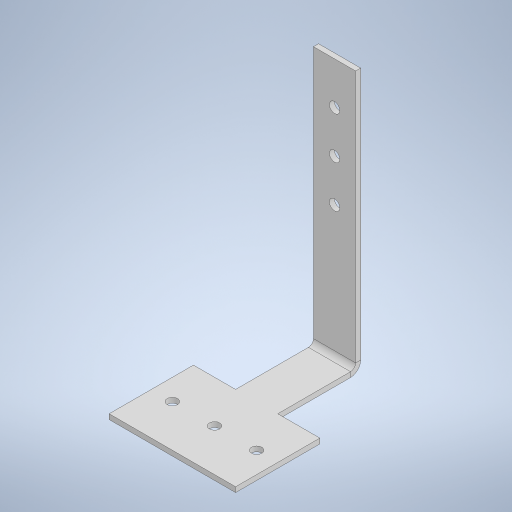
# Autodesk Inventor part: Flexible Bracket
Saved by Autodesk Inventor 2023 (Build 270158000, 158)
## iProperties
Created: 2022-07-19
Part Number: Flexible Bracket
Material: Generic
Document SubType Name: Sheet Metal
Designer: EricPaul
Density: 1 g/cm^3
Sheet Metal Rule: Default
Appearance: Default
Author: EricPaul
Autodesk Inventor part; units mm, degrees
ref_plane "YZ Plane" through (0, 0, 0) normal (1, 0, 0) x (0, 1, 0)
ref_plane "XZ Plane" through (0, 0, 0) normal (0, 1, 0) x (-1, 0, 0)
ref_plane "XY Plane" through (0, 0, 0) normal (0, 0, 1) x (1, 0, 0)
sketch "Sketch7" plane through (0, 0, 0) normal (0, 1, 0) x (-1, 0, 0)
  line L0 (12.7, 25.4) -> (-12.7, 25.4)
  line L1 (-12.7, 25.4) -> (-12.7, -228.6)
  line L2 (-12.7, -228.6) -> (12.7, -228.6)
  line L3 (12.7, -228.6) -> (12.7, 25.4)
  line L4 (12.7, 25.4) -> (-12.7, -228.6) construction
  line L5 (-12.7, 25.4) -> (12.7, -228.6) construction
  line L6 (0, -279.4) -> (0, 76.2)
  line L7 (-38.1, -25.4) -> (-38.1, 25.4)
  line L8 (-38.1, 25.4) -> (38.1, 25.4)
  line L9 (38.1, 25.4) -> (38.1, -25.4)
  line L10 (38.1, -25.4) -> (-38.1, -25.4)
  line L11 (-38.1, -25.4) -> (38.1, 25.4) construction
  line L12 (-38.1, 25.4) -> (38.1, -25.4) construction
  point P0 (0, 0)
  point P1 (0, -101.6)
  point P2 (0, 25.4)
  dimension "d17" = 25.4
  dimension "d18" = 254
  dimension "d19" = 25.4
  dimension "d38" = 76.2
  dimension "d39" = 50.8
  measures "d17" distance of L0.start L0.end
  measures "d18" distance of L1.end L0.end
  measures "d19" distance from line of L0 point (0, 0)
  measures "d38" distance of L7.end L8.end
  measures "d39" distance of L7.start L7.end
extrude "Plate3" add sketch "Sketch7" along normal blind 3.048
sketch "Sketch8" plane through (0, 3.048, 0) normal (0, 1, 0) x (1, 0, 0)
  line L0 (0, 279.4) -> (0, -76.2) projected
  line L1 (-12.7, 228.6) -> (12.7, 228.6) projected
  point P0 (0, 0)
  point P1 (0, 0)
  point P2 (0, 203.2)
  point P3 (0, 152.4)
  point P4 (0, 177.8)
  point P5 (-25.4, 0)
  point P6 (25.4, 0)
  dimension "d21" = 25.4
  dimension "d22" = 50.8
  dimension "d23" = 76.2
  dimension "d40" = 25.4
  dimension "d41" = 25.4
  constraints: 3 point on line, 1 coincident
  measures "d21" distance from line of point (0, 203.2) L1
  measures "d22" distance from line of point (0, 177.8) L1
  measures "d23" distance from line of point (0, 152.4) L1
  measures "d40" distance of point (-25.4, 0) point (0, 0)
  measures "d41" distance of point (25.4, 0) point (0, 0)
hole "Hole1" at (0, 3.048, 0) at (0, 3.048, -203.2) at (0, 3.048, -152.4) at (0, 3.048, -177.8) at (-25.4, 3.048, 0) at (25.4, 3.048, 0) direction (0, -1, 0) diameter 6.35 end through all
sketch "Sketch9" plane through (0, 3.048, 0) normal (0, 1, 0) x (1, 0, 0)
  line L0 (-12.7, 25.4) -> (-12.7, 228.6) projected
  line L1 (12.7, 228.6) -> (12.7, 25.4) projected
  line L2 (-12.7, 76.2) -> (12.7, 76.2)
  point P0 (0, 0)
  point P1 (-12.7, -25.4)
  point P2 (12.7, -25.4)
  dimension "d31" = 76.2
  constraints: 2 end point, 2 point on line, 1 perpendicular
  measures "d31" distance from line of point (0, 0) L2
fold "Fold3" angle 90 bend radius 3.048 thickness 3.048 k factor 0.44 line from (-12.7, 3.048, -76.2) to (12.7, 3.048, -76.2) line at bend end moving side (0, 0, -1) folds toward (0, 1, 0)
equation "\"d29\" = Thickness"
equation "\"d20\" = Thickness"
equation "\"d31\" = SupportDistance"
equation "\"d32\" = BendReliefWidth"
equation "\"d33\" = BendReliefDepth"
equation "\"d34\" = MinimumRemnant"
equation "\"d35\" = TransitionRadius"
equation "\"d37\" = BendRadius"
equation "\"BendRadius\" = Thickness"
equation "\"BendReliefWidth\" = Thickness"
equation "\"BendReliefDepth\" = 0.5 * Thickness"
equation "\"CornerReliefSize\" = 4 * Thickness"
equation "\"MinimumRemnant\" = 2 * Thickness"
equation "\"TransitionRadius\" = BendRadius"
equation "\"JacobiRadiusSize\" = BendRadius"
equation "\"GapSize\" = Thickness"
equation "\"SupportDistance\" = 76.2"
equation "\"Thickness\" = 3.048"
body "Solid3"
